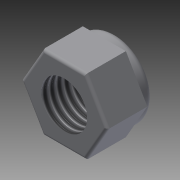
# Autodesk Inventor part: dadoAutobloccante
Saved by Autodesk Inventor 2014 SP2 (Build 180246200, 246)
## iProperties
Created: 2019-05-12
Part Number: dadoAutobloccante
Material: Generic
Document SubType Name: Modeling
Designer: GauchoHP
Density: 1 g/cm^3
Appearance: Default
Author: GauchoHP
Autodesk Inventor part; units mm, degrees
ref_plane "YZ Plane" through (0, 0, 0) normal (1, 0, 0) x (0, 1, 0)
ref_plane "XZ Plane" through (0, 0, 0) normal (0, 1, 0) x (-1, 0, 0)
ref_plane "XY Plane" through (0, 0, 0) normal (0, 0, 1) x (1, 0, 0)
sketch "Sketch1" plane through (0, 0, 0) normal (0, 1, 0) x (-1, 0, 0)
  line L0 (3.7528, 6.5) -> (7.5056, 0)
  line L1 (7.5056, 0) -> (3.7528, -6.5)
  line L2 (3.7528, -6.5) -> (-3.7528, -6.5)
  line L3 (-3.7528, -6.5) -> (-7.5056, 0)
  line L4 (-7.5056, 0) -> (-3.7528, 6.5)
  line L5 (-3.7528, 6.5) -> (3.7528, 6.5)
  circle A0 centre (0, 0) radius 4
  dimension "d0" = 13
  dimension "d1" = 8
  constraints: 12 end point, 2 coincident, 1 centre point, 13 other
  measures "d0" distance between parallel lines of L5 L2
  measures "d1" diameter of A0
extrude "Extrusion1" add sketch "Sketch1" along normal blind 7
thread "Thread1" size "M8x1.25" class "6H" standard "ANSI Metric M Profile" full length
sketch "Sketch2" plane through (0, 7, 0) normal (0, 1, 0) x (1, 0, 0)
  circle A0 centre (0, 0) radius 4 projected
  circle A1 centre (0, 0) radius 6.5
  constraints: 1 centre point, 1 coincident
extrude "Extrusion2" add sketch "Sketch2" along normal blind 2
fillet "Fillet1" radius 0.999 2 edges at (-6.5, 9, 0) (-4, 9, 0)
fillet "Fillet2" radius 0.5 6 edges at (0, 0, 6.5) (5.6292, 0, 3.25) (5.6292, 0, -3.25) (0, 0, -6.5) (-5.6292, 0, -3.25) (-5.6292, 0, 3.25)
body "Solid1"
